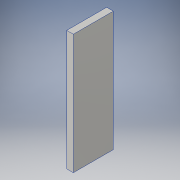
# Autodesk Inventor part: bottomOfShooter
Saved by Autodesk Inventor 2016 SP1 (Build 200210100, 210)
## iProperties
Created: 2016-02-08
Part Number: bottomOfShooter
Material: Aluminum 6061
Document SubType Name: Modeling
Designer: steele
Density: 2.7 g/cm^3
Appearance: Aluminum - Flat
Author: steele
Autodesk Inventor part; units mm, degrees
ref_plane "YZ Plane" through (0, 0, 0) normal (1, 0, 0) x (0, 1, 0)
ref_plane "XZ Plane" through (0, 0, 0) normal (0, 1, 0) x (-1, 0, 0)
ref_plane "XY Plane" through (0, 0, 0) normal (0, 0, 1) x (1, 0, 0)
sketch "Sketch1" plane through (0, 0, 0) normal (0, 0, 1) x (1, 0, 0)
  line L0 (-3.175, -57.15) -> (3.175, -57.15)
  line L1 (3.175, -57.15) -> (3.175, 57.15)
  line L2 (3.175, 57.15) -> (-3.175, 57.15)
  line L3 (-3.175, 57.15) -> (-3.175, -57.15)
  line L4 (-3.175, -57.15) -> (3.175, 57.15) construction
  line L5 (3.175, -57.15) -> (-3.175, 57.15) construction
  point P0 (0, 0)
  dimension "d11" = 6.35
  dimension "d12" = 114.3
  constraints: 12 end point, 2 midpoint, 2 parallel, 1 horizontal, 1 perpendicular
  measures "d11" distance of L1.end L2.end
  measures "d12" distance of L2.end L0.start
extrude "Extrusion5" add sketch "Sketch1" along normal mid plane 38.1
equation "\"d12\" = length"
equation "\"d17\" = longSide"
equation "\"width\" = 19.05"
equation "\"longSide\" = 38.1"
equation "\"length\" = 114.3"
body "Solid3"
